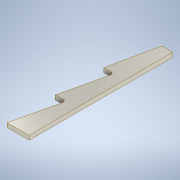
# Autodesk Inventor part: spikyboi
Saved by Autodesk Inventor 2020 (Build 240168000, 168)
## iProperties
Created: 2020-05-04
Part Number: spikyboi
Material: Titanium
Document SubType Name: Modeling
Designer: marah
Density: 4.51 g/cm^3
Appearance: Titanium
Mass: 0.555179 g
Surface Area: 3.24646 cm^2
Volume: 0.1231 cm^3
Author: marah
Autodesk Inventor part; units mm, degrees
ref_plane "YZ Plane" through (0, 0, 0) normal (1, 0, 0) x (0, 1, 0)
ref_plane "XZ Plane" through (0, 0, 0) normal (0, 1, 0) x (-1, 0, 0)
ref_plane "XY Plane" through (0, 0, 0) normal (0, 0, 1) x (1, 0, 0)
sketch "Sketch1" plane through (0, 0, 0) normal (0, 1, 0) x (-1, 0, 0)
  line L0 (0, 0) -> (0, 33)
  line L1 (0, 33) -> (5, 33)
  line L2 (0, 0) -> (0, 11) construction
  line L3 (0, 11) -> (0, 22) construction
  line L4 (0, 22) -> (0, 33) construction
  line L5 (0, 22) -> (5, 22) construction
  line L6 (0, 11) -> (5, 11) construction
  line L7 (5, 33) -> (2.5, 22)
  line L8 (2.5, 22) -> (5, 22)
  line L9 (5, 22) -> (2.5, 11)
  line L10 (4.8494, 11) -> (2.5, 11)
  line L11 (0, 0) -> (5, 0) construction
  line L12 (4.8494, 11) -> (2.5, 0)
  line L13 (0, 0) -> (2.5, 0)
  dimension "d0" = 33
  dimension "d1" = 5
  dimension "d13" = 11
  dimension "d14" = 11
  dimension "d15" = 5
  dimension "d16" = 5
  dimension "d17" = 5
  constraints: 28 end point, 4 collinear, 3 midpoint, 3 point on line, 2 horizontal, 1 parallel, 1 perpendicular, 1 vertical
  measures "d0" distance of L0.start L0.end
  measures "d1" distance of L0.end L1.end
  measures "d13" distance of L0.start L2.end
  measures "d14" distance of L2.end L3.end
  measures "d15" distance of L3.end L5.end
  measures "d16" distance of L2.end L6.end
  measures "d17" distance of L0.start L11.end
extrude "Extrusion1" add sketch "Sketch1" along normal blind 1
fillet "Fillet1" radius 0.5 2 edges at (-2.5, 0.5, 11) (-2.5, 0.5, 22)
body "Solid1"
